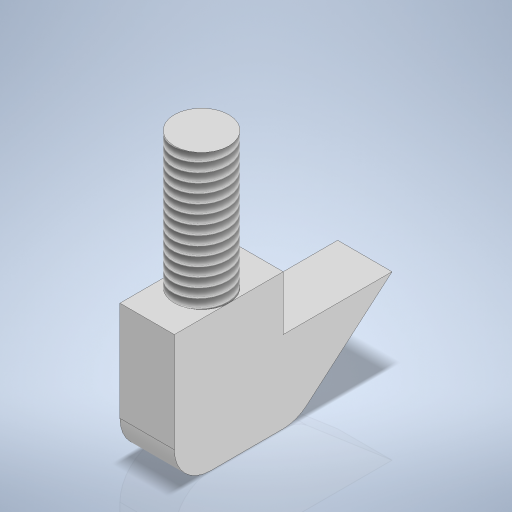
# Autodesk Inventor part: 1 part 8
Saved by Autodesk Inventor 2024 (Build 280153000, 153)
## iProperties
Created: 2024-07-24
Part Number: 1 part 8
Material: Generisch
Document SubType Name: Modeling
Designer: ffogue
Density: 1 g/cm^3
Appearance: Vorgabe
Author: ffogue
Autodesk Inventor part; units mm, degrees
ref_plane "YZ Plane" through (0, 0, 0) normal (1, 0, 0) x (0, 1, 0)
ref_plane "XZ Plane" through (0, 0, 0) normal (0, 1, 0) x (-1, 0, 0)
ref_plane "XY Plane" through (0, 0, 0) normal (0, 0, 1) x (1, 0, 0)
sketch "Skizze1" plane through (0, 0, 0) normal (1, 0, 0) x (0, 1, 0)
  line L0 (0, 0) -> (0, -5.5)
  line L1 (2, -7.5) -> (6, -7.5)
  line L2 (7.3, -7.0199) -> (12, -3)
  line L3 (12, -3) -> (6, -3)
  line L4 (6, -3) -> (6, 0)
  line L5 (6, 0) -> (1.5, 0)
  line L6 (1.5, 0) -> (0, 0)
  arc A0 (0, -5.5) -> (2, -7.5) centre (2, -5.5) ccw
  arc A1 (6, -7.5) -> (7.3, -7.0199) centre (6, -5.5) ccw
  dimension "d3" = 3
  dimension "d4" = 6
  dimension "d8" = 2
  dimension "d9" = 6
  dimension "d10" = 7.5
  constraints: 15 end point, 4 point on circle, 4 tangent, 3 perpendicular, 2 centre point, 2 coincident, 1 equal radius, 1 parallel, 1 point on line, 1 vertical, 1 vertical alignment
  measures "d3" distance of L3.end L4.end
  measures "d4" distance from line of L2.end L4
  measures "d8" radius of A0
  measures "d9" distance of L4.end point (0, 0)
  measures "d10" distance from line of L1.end L5
extrude "Extrusion1" add sketch "Skizze1" along normal mid plane 3
sketch "Skizze2" plane through (-1.5, 0, 0) normal (0, 0, 1) x (1, 0, 0)
  circle A0 centre (1.5, 3) radius 1.5
  line L0 (0, 0) -> (3, 0) projected
  point P0 (1.5, 0)
  point P1 (1.5, 0)
  point P2 (1.5, 0)
  dimension "d13" = 3
  dimension "d14" = 3
  constraints: 2 midpoint, 1 centre point, 1 vertical alignment
  measures "d13" diameter of A0
  measures "d14" distance of point (1.5, 0) A0.centre
extrude "Extrusion2" add sketch "Skizze2" along normal blind 7.5
thread "Gewinde1" size "M3x0.5" class "6g" standard "ISO Metric profile" length 11
